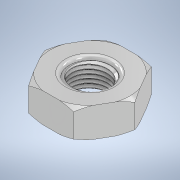
# Autodesk Inventor part: Tca. Hex estandar
Saved by Autodesk Inventor 2020 (Build 240168000, 168)
## iProperties
Created: 2020-09-17
Part Number: Tca. Hex estandar
Material: Aluminum 6061-AHC
Document SubType Name: Modeling
Designer: aaron
Density: 2.7 g/cm^3
Appearance: Aluminum - Polished
Author: aaron
Autodesk Inventor part; units mm, degrees
ref_plane "YZ Plane" through (0, 0, 0) normal (1, 0, 0) x (0, 1, 0)
ref_plane "XZ Plane" through (0, 0, 0) normal (0, 1, 0) x (-1, 0, 0)
sketch "Sketch1" plane through (0, 0, 0) normal (0, 1, 0) x (-1, 0, 0)
  line L0 (-15.5886, 0) -> (-7.7943, 13.5001)
  line L1 (-7.7943, 13.5001) -> (7.7943, 13.5001)
  line L2 (7.7943, 13.5001) -> (15.5886, 0)
  line L3 (15.5886, 0) -> (7.7943, -13.5001)
  line L4 (7.7943, -13.5001) -> (-7.7943, -13.5001)
  line L5 (-7.7943, -13.5001) -> (-15.5886, 0)
  point P0 (0, 0)
  point P1 (0, 0)
  point P2 (0, 0)
  dimension "d0" = 27.0002
  constraints: 12 end point, 2 coincident, 1 horizontal alignment, 13 other
  measures "d0" distance between parallel lines of L1 L4
extrude "Extrusion1" add sketch "Sketch1" against normal blind 10.2362
hole "Hole1" at (0, 0, 0) direction (0, -1, 0) diameter 14.351 end through all thread size "5/8-18 UNF" class "3B" standard "ANSI Unified Screw Threads"
fillet "Fillet1" radius 1.27 1 edges at (0, 0, -7.1755)
fillet "Fillet2" radius 1.27 1 edges at (0, -10.2362, -7.1755)
thread "Thread1" size "5/8-18 UNF" class "2B" standard "ANSI Unified Screw Threads" full length
sketch "Sketch3" plane through (0, -1.27, 0) normal (1, 0, 0) x (0, 0, 1)
  line L0 (7.1755, 0) -> (7.1755, 7.6962)
  line L1 (7.1755, 7.6962) -> (6.1292, 7.6962)
  line L2 (6.1292, 7.6962) -> (6.1292, 0)
  line L3 (6.1292, 0) -> (7.1755, 0)
  line L4 (0, -3.6398) -> (0, 11.0672) projected
  constraints: 8 end point
revolve "Revolution1" add sketch "Sketch3" angle 360 about axis through (0, -1.27, 0) along (0, -1, 0) separate body
sketch "Sketch2" plane through (0, -1.27, 7.1755) normal (-1, 0, 0) x (0, -1, 0)
  line L0 (-0.8233, -0.0715) -> (-0.7057, -0.0715) construction
  line L1 (0.1175, -0.9751) -> (-0.0001, -1.201) construction
  line L2 (-1.4112, -1.201) -> (-1.5288, -0.9751) construction
  line L3 (-0.5881, -0.0715) -> (-0.7057, 0.1544) construction
  line L4 (-0.7057, 0.1544) -> (-0.8233, -0.0715) construction
  line L5 (-1.4112, -1.201) -> (-1.2936, -0.9751) construction
  line L6 (-0.5881, -0.0715) -> (-0.1177, -0.9751)
  line L7 (-1.5288, -0.9751) -> (-1.2936, -0.9751) construction
  arc A0 (-1.5288, -0.9751) -> (-1.4112, -1.0465) centre (-1.4112, -0.9139) ccw construction
  line L8 (0.1175, -0.9751) -> (-0.1177, -0.9751) construction
  line L9 (-1.4112, -1.201) -> (-1.4112, -0.9751) construction
  line L10 (-0.0001, -1.201) -> (-0.0001, -0.9751) construction
  line L11 (-0.7057, 0.1544) -> (-0.7057, -0.0002) construction
  line L12 (-1.4112, -1.0465) -> (-0.0001, -1.0465)
  arc A1 (-1.4112, -1.0465) -> (-1.2936, -0.9751) centre (-1.4112, -0.9139) ccw
  line L13 (-0.1177, -0.9751) -> (-0.0001, -1.201) construction
  line L14 (-1.2936, -0.9751) -> (-0.8233, -0.0715)
  line L15 (-0.0001, -0.0002) -> (-0.0001, 0.0177)
  line L16 (-0.0001, 0.0177) -> (-0.0001, -0.0002)
  line L17 (-0.0001, -0.0002) -> (0.0334, -0.0002)
  arc A2 (-0.1177, -0.9751) -> (-0.0001, -1.0465) centre (-0.0001, -0.9139) ccw
  arc A3 (-0.0001, -1.0465) -> (0.1175, -0.9751) centre (-0.0001, -0.9139) ccw construction
  arc A4 (-0.7057, -0.0002) -> (-0.8233, -0.0715) centre (-0.7057, -0.1327) ccw
  arc A5 (-0.5881, -0.0715) -> (-0.7057, -0.0002) centre (-0.7057, -0.1327) ccw
  line L18 (-0.7057, -0.0002) -> (-0.7057, -0.0715) construction
  line L19 (-0.7057, -0.0715) -> (-0.5881, -0.0715) construction
  dimension "d14" = 55
  dimension "d15" = 0.2259
  dimension "d16" = 0.2259
  dimension "Sketch2_ThreadOffset" = 0
  dimension "Sketch2_MajorRadius" = 1.0463
  dimension "d19" = 1.4111
  dimension "Sketch2_MinorRadius" = 0
  constraints: 40 end point, 12 point on circle, 10 parallel, 8 tangent, 6 centre point, 6 collinear, 2 midpoint, 2 point on line, 1 horizontal, 1 perpendicular, 3 other
  measures "d14" angle of L6 L14
  measures "d15" distance of L3.end L0.end
  measures "d16" distance of L1.end L10.end
  measures "Sketch2_ThreadOffset" distance between parallel lines of L15 L10
  measures "Sketch2_MajorRadius" distance from line of L12 L15.start
  measures "d19" distance from line of L1.end L9
  measures "Sketch2_MinorRadius" distance edge to line of A5 L17
coil "Coil1" sketch "Sketch2" operation cut axis through (0, -1.27, 0) along (0, -1, 0) pitch 1.4125 turns 7.446553 hand right bodies 2
ref_plane "Work Plane1" through (7.7943, 0, -13.5001) normal (-0.8660254, 0, -0.5) x (0, -1, 0)
sketch "Sketch5" plane through (7.7943, 0, -13.5001) normal (-0.8660254, 0, -0.5) x (0, -1, 0)
  line L0 (0, 0) -> (0, 7.7943) projected
  line L1 (0, 0) -> (0, 1.7598)
  line L2 (0, 1.7598) -> (1.016, 0)
  line L3 (1.016, 0) -> (0, 0)
  line L4 (0, 0) -> (0, 7.7943) construction
  line L5 (0, 0) -> (10.2362, 0) construction
  line L6 (10.2362, 7.7943) -> (10.2362, 0) construction
  line L7 (0, 7.7943) -> (10.2362, 7.7943) construction
  line L8 (5.1181, 0) -> (5.1181, 7.7943) construction
  line L9 (10.2362, 0) -> (10.2362, 7.7943)
  line L10 (10.2362, 0) -> (10.2362, 1.7598)
  line L11 (10.2362, 1.7598) -> (9.2202, 0)
  line L12 (9.2202, 0) -> (10.2362, 0)
  line L13 (12.2834, 15.5886) -> (-2.0472, 15.5886) projected
  point P0 (0, 15.5886)
  dimension "d34" = 60
  dimension "d35" = 1.016
  constraints: 16 end point, 4 symmetric about line, 2 midpoint, 2 point on line, 1 perpendicular
  measures "d34" angle of L2 L3
  measures "d35" distance of L2.end L0.start
revolve "Revolution2" cut sketch "Sketch5" angle 360 about axis through (0, -10, 0) along (0, 1, 0) bodies 1
equation "\"d14\" = d21"
equation "\"d15\" = 0.160083 * Sketch2_Pitch"
equation "\"d16\" = 0.160083 * Sketch2_Pitch"
equation "\"d19\" = Sketch2_Pitch"
equation "\"d21\" = 55deg"
equation "\"Sketch2_Pitch\" = 1.41111"
body "Solid1"
body "Solid2"
